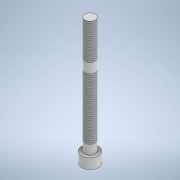
# Autodesk Inventor part: M8x80_threaded
Saved by Autodesk Inventor 2020.3 (Build 243373000, 373)
## iProperties
Created: 2021-03-23
Part Number: M8x80_threaded
Material: Ogólny
Document SubType Name: Modeling
Designer: patry
Density: 1 g/cm^3
Appearance: Domyślna
Author: patry
Autodesk Inventor part; units mm, degrees
ref_plane "YZ Plane" through (0, 0, 0) normal (1, 0, 0) x (0, 1, 0)
ref_plane "XZ Plane" through (0, 0, 0) normal (0, 1, 0) x (-1, 0, 0)
ref_plane "XY Plane" through (0, 0, 0) normal (0, 0, 1) x (1, 0, 0)
sketch "Szkic1" plane through (0, 0, 0) normal (0, 1, 0) x (-1, 0, 0)
  circle A0 centre (0, 0) radius 6.5
  line L0 (1.7321, 3) -> (3.4641, 0)
  line L1 (3.4641, 0) -> (1.7321, -3)
  line L2 (1.7321, -3) -> (-1.7321, -3)
  line L3 (-1.7321, -3) -> (-3.4641, 0)
  line L4 (-3.4641, 0) -> (-1.7321, 3)
  line L5 (-1.7321, 3) -> (1.7321, 3)
  circle A1 centre (0, 0) radius 4
  dimension "d0" = 13
  dimension "d1" = 6
  dimension "d12" = 8
  constraints: 12 end point, 3 coincident, 2 centre point, 13 other
  measures "d0" diameter of A0
  measures "d1" distance between parallel lines of L2 L5
  measures "d12" diameter of A1
extrude "Wyciągnięcie proste1" add sketch "Szkic1" along normal blind 4 contours A0 | L0 L1 L2 L3 L4 L5 | A1
extrude "Wyciągnięcie proste2" add sketch "Szkic1" against normal blind 4 contours A0 | A1
sketch "Szkic2" plane through (0, 4, 0) normal (0, 1, 0) x (1, 0, 0)
  circle A0 centre (0, 0) radius 4
  dimension "d7" = 8
  constraints: 1 centre point, 1 coincident
  measures "d7" diameter of A0
extrude "Wyciągnięcie proste3" add sketch "Szkic2" along normal blind 90
thread "Gwint1" size "M8x1.25" class "6g" standard "ANSI Metric M Profile" length 48 offset 35
thread "Gwint2" size "M8x1.25" class "6g" standard "ANSI Metric M Profile" length 28
